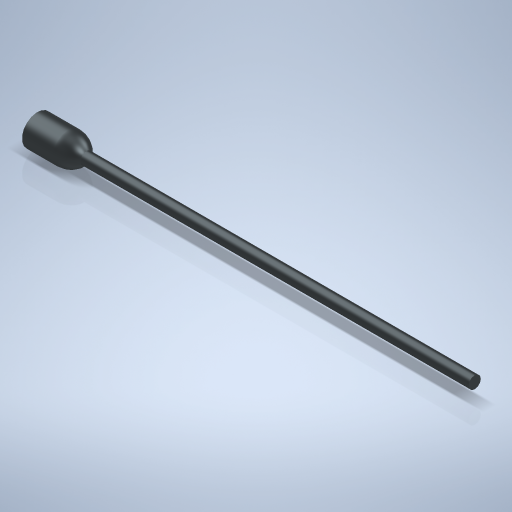
# Autodesk Inventor part: rod
Saved by Autodesk Inventor 2024 (Build 280153000, 153)
## iProperties
Created: 2024-04-24
Part Number: rod
Material: Eisen, Grau
Document SubType Name: Modeling
Designer: ffogue
Density: 7.15 g/cm^3
Appearance: Eisen - Grau
Author: ffogue
Autodesk Inventor part; units mm, degrees
ref_plane "YZ Plane" through (0, 0, 0) normal (1, 0, 0) x (0, 1, 0)
ref_plane "XZ Plane" through (0, 0, 0) normal (0, 1, 0) x (-1, 0, 0)
ref_plane "XY Plane" through (0, 0, 0) normal (0, 0, 1) x (1, 0, 0)
sketch "Skizze1" plane through (0, 0, 0) normal (0, 0, 1) x (1, 0, 0)
  line L0 (0, 0) -> (57, 0)
  line L1 (0, 0) -> (0, 2)
  line L2 (0, 2) -> (4, 2)
  arc A0 (6.4, 0.8) -> (4, 2) centre (4, -1) ccw
  line L3 (6.4, 0.8) -> (57, 0.8)
  line L4 (57, 0.8) -> (57, 0)
  dimension "d0" = 4
  dimension "d1" = 1.6
  dimension "d2" = 3
  dimension "d3" = 4
  dimension "d4" = 57
  constraints: 11 end point, 2 horizontal, 2 perpendicular, 2 point on circle, 1 centre point, 1 tangent, 1 vertical
  measures "d0" diameter of L1.end L0
  measures "d1" diameter of L3 L0
  measures "d2" radius of A0
  measures "d3" distance from line of L1 L2.end
  measures "d4" distance between parallel lines of L1 L4
revolve "Umdrehung1" add sketch "Skizze1" angle 360 about axis through (0, 0, 0) along (1, 0, 0)
shell "Wandung1" thickness 0.25 removed faces 1 at (0, 0.6473, -0.1595)
